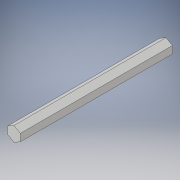
# Autodesk Inventor part: Sanded Hex Rod
Saved by Autodesk Inventor 2018 (Build 220112000, 112)
## iProperties
Created: 2019-01-13
Part Number: Sanded Hex Rod
Material: Generic
Document SubType Name: Modeling
Designer: Gabriel
Density: 1 g/cm^3
Appearance: Default
Author: Gabriel
Autodesk Inventor part; units mm, degrees
ref_plane "YZ Plane" through (0, 0, 0) normal (1, 0, 0) x (0, 1, 0)
ref_plane "XZ Plane" through (0, 0, 0) normal (0, 1, 0) x (-1, 0, 0)
ref_plane "XY Plane" through (0, 0, 0) normal (0, 0, 1) x (1, 0, 0)
sketch "Sketch1" plane through (0, 0, 0) normal (0, 0, 1) x (1, 0, 0)
  line L0 (-15.6518, 12.7321) -> (-8.8412, 16.685)
  line L1 (-15.6518, 12.7321) -> (-18.8393, 18.2241)
  line L2 (-18.8393, 10.8821) -> (-25.1977, 14.5531)
  line L3 (-25.1977, 14.5531) -> (-25.1977, 21.8951)
  line L4 (-25.1977, 21.8951) -> (-18.8393, 25.5661)
  line L5 (-18.8393, 25.5661) -> (-12.481, 21.8951)
  line L6 (-12.481, 21.8951) -> (-12.481, 14.5531)
  line L7 (-12.481, 14.5531) -> (-18.8393, 10.8821)
  dimension "d5" = 6.35
  constraints: 16 end point, 1 coincident, 13 other
  measures "d5" distance of L0.start L1.end
extrude "Extrusion1" add sketch "Sketch1" along normal blind 152.4
body "Solid1"
